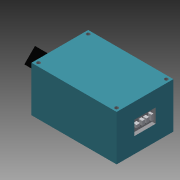
# Autodesk Inventor part: motor
Saved by Autodesk Inventor 2015 (Build 190159000, 159)
## iProperties
Created: 2014-11-09
Part Number: motor
Material: Generic
Document SubType Name: Modeling
Designer: ericd_000
Density: 1 g/cm^3
Appearance: Default
Author: ericd_000
Autodesk Inventor part; units mm, degrees
ref_plane "YZ Plane" through (0, 0, 0) normal (1, 0, 0) x (0, 1, 0)
ref_plane "XZ Plane" through (0, 0, 0) normal (0, 1, 0) x (-1, 0, 0)
ref_plane "XY Plane" through (0, 0, 0) normal (0, 0, 1) x (1, 0, 0)
sketch "Sketch1" plane through (0, 0, 0) normal (0, 0, 1) x (1, 0, 0)
  line L0 (-60, 40) -> (60, 40)
  line L1 (60, 40) -> (60, -40)
  line L2 (60, -40) -> (-60, -40)
  line L3 (-60, -40) -> (-60, 40)
  point P0 (0, 0)
  point P1 (-60, 0)
  point P2 (0, 40)
  dimension "d0" = 120
  dimension "d1" = 80
  constraints: 8 end point, 2 midpoint, 2 parallel, 1 horizontal, 1 horizontal alignment, 1 perpendicular, 1 vertical alignment
  measures "d0" distance of L0.start L0.end
  measures "d1" distance of L2.end L0.start
extrude "Extrusion1" add sketch "Sketch1" along normal blind 64
sketch "Sketch4" plane through (-60, -40, 0) normal (-1, 0, 0) x (0, 0, 1)
  circle A0 centre (32, 40) radius 15
  line L0 (0, 0) -> (0, 80) projected
  line L1 (0, 80) -> (64, 80) projected
  point P0 (0, 40)
  point P1 (0, 40)
  point P2 (32, 80)
  dimension "d12" = 30
  constraints: 2 midpoint, 1 centre point, 1 horizontal alignment, 1 vertical alignment
  measures "d12" diameter of A0
extrude "Extrusion2" add sketch "Sketch4" along normal blind 35
sketch "Sketch7" plane through (-95, 0, 32) normal (-1, 0, 0) x (0, 0, 1)
  circle A0 centre (0, 0) radius 15 projected
  line L0 (0, 15) -> (15, 0)
  line L1 (0, -15) -> (15, 0)
  line L2 (0, -15) -> (-15, 0)
  line L3 (0, 15) -> (-15, 0)
  point P0 (-32, 0)
  constraints: 8 end point, 4 point on circle, 3 perpendicular
extrude "Extrusion3" cut sketch "Sketch7" against normal blind 30 contours L0 A0 | A0 L1 | L3 A0 | A0 L2
sketch "Sketch8" plane through (60, -40, 0) normal (1, 0, 0) x (0, 0, -1)
  line L0 (-42, 25) -> (-22, 25)
  line L1 (-22, 25) -> (-22, 55)
  line L2 (-22, 55) -> (-42, 55)
  line L3 (-42, 55) -> (-42, 25)
  line L4 (0, 0) -> (-64, 0) projected
  line L5 (-64, 0) -> (-64, 80) projected
  line L6 (-30, 33) -> (-34, 33)
  line L7 (-34, 33) -> (-34, 28)
  line L8 (-34, 28) -> (-30, 28)
  line L9 (-30, 28) -> (-30, 33)
  line L10 (-29, 40) -> (-35, 40)
  line L11 (-35, 40) -> (-35, 36)
  line L12 (-35, 36) -> (-29, 36)
  line L13 (-29, 36) -> (-29, 40)
  line L14 (-29, 46) -> (-35, 46)
  line L15 (-35, 46) -> (-35, 42)
  line L16 (-35, 42) -> (-29, 42)
  line L17 (-29, 42) -> (-29, 46)
  line L18 (-36, 49) -> (-28, 49)
  line L19 (-28, 49) -> (-28, 52)
  line L20 (-28, 52) -> (-36, 52)
  line L21 (-36, 52) -> (-36, 49)
  point P0 (0, 40)
  point P1 (-32, 25)
  point P2 (-32, 0)
  point P3 (-42, 40)
  point P4 (-64, 40)
  point P5 (-32, 28)
  point P6 (-32, 36)
  point P7 (-32, 42)
  point P8 (-32, 52)
  point P9 (-32, 55)
  dimension "d17" = 30
  dimension "d18" = 20
  dimension "d19" = 5
  dimension "d20" = 4
  dimension "d21" = 4
  dimension "d22" = 6
  dimension "d23" = 6
  dimension "d24" = 4
  dimension "d27" = 3
  dimension "d28" = 8
  dimension "d29" = 3
  dimension "d30" = 2
  dimension "d31" = 3
  dimension "d32" = 3
  constraints: 40 end point, 10 parallel, 9 midpoint, 5 horizontal, 5 perpendicular, 5 vertical alignment, 1 horizontal alignment
  measures "d17" distance of L2.end L0.start
  measures "d18" distance of L1.end L2.end
  measures "d19" distance of L6.end L7.end
  measures "d20" distance of L7.end L8.end
  measures "d21" distance of L10.end L11.end
  measures "d22" distance of L10.start L10.end
  measures "d23" distance of L14.start L14.end
  measures "d24" distance of L14.end L15.end
  measures "d27" distance of L20.end L18.start
  measures "d28" distance of L18.start L18.end
  measures "d29" distance between parallel lines of L12 L6
  measures "d30" distance between parallel lines of L16 L10
  measures "d31" distance between parallel lines of L18 L14
  measures "d32" distance between parallel lines of L0 L8
extrude "Extrusion4" cut sketch "Sketch8" against normal blind 5
sketch "Sketch9" plane through (0, 0, 64) normal (0, 0, 1) x (1, 0, 0)
  circle A0 centre (-55, 35) radius 2.5
  line L0 (-60, 40) -> (-60, -40) projected
  line L1 (60, 40) -> (-60, 40) projected
  circle A1 centre (55, 35) radius 2.5
  circle A2 centre (-55, -35) radius 2.5
  circle A3 centre (55, -35) radius 2.5
  point P0 (0, 0)
  dimension "d35" = 5
  dimension "d36" = 5
  dimension "d37" = 5
  dimension "d40" = 110
  dimension "d43" = 70
  constraints: 4 centre point, 1 horizontal, 1 vertical, 6 other
  measures "d35" diameter of A0
  measures "d36" distance from line of L0 A0.centre
  measures "d37" distance from line of L1 A0.centre
  measures "d40" distance of A0.centre A1.centre
  measures "d43" distance of A0.centre A2.centre
extrude "Extrusion5" cut sketch "Sketch9" against normal blind 5
body "Solid1"
